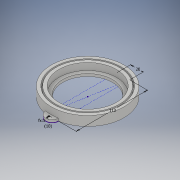
# Autodesk Inventor part: Cap
Saved by Autodesk Inventor 2018 (Build 220112000, 112)
## iProperties
Created: 2017-06-25
Part Number: Cap
Material: Generic
Document SubType Name: Modeling
Designer: Soichi
Density: 1 g/cm^3
Appearance: Default
Author: Soichi
Autodesk Inventor part; units mm, degrees
ref_plane "YZ Plane" through (0, 0, 0) normal (1, 0, 0) x (0, 1, 0)
ref_plane "XZ Plane" through (0, 0, 0) normal (0, 1, 0) x (-1, 0, 0)
ref_plane "XY Plane" through (0, 0, 0) normal (0, 0, 1) x (1, 0, 0)
sketch "Sketch1" plane through (0, 0, 0) normal (0, 0, 1) x (1, 0, 0)
  circle A0 centre (0, 0) radius 57.5
  dimension "d0" = 115
  constraints: 1 centre point, 1 coincident
  measures "d0" diameter of A0
sketch "Sketch2" plane through (0, 0, 0) normal (1, 0, 0) x (0, 1, 0)
  line L0 (57.5, 0) -> (-57.5, 0) construction
  line L1 (-57.5, 0) -> (-57.5, 15)
  line L2 (-57.5, 15) -> (-39.5, 15)
  line L3 (-39.5, 15) -> (-39.5, 11)
  line L4 (-57.5, 0) -> (-52.5, 0)
  line L5 (-52.5, 0) -> (-52.5, 8)
  line L6 (-52.5, 8) -> (-50.42, 8)
  line L7 (-50.42, 8) -> (-50.42, 0)
  line L8 (-50.42, 0) -> (-45.42, 0)
  line L9 (-50.42, 0) -> (-45.42, 0) construction
  line L10 (-45.42, 0) -> (-45.42, 11)
  line L11 (-45.42, 11) -> (-39.5, 11)
  point P0 (0, 0)
  dimension "d1" = 15
  dimension "d3" = 4
  dimension "d4" = 90
  dimension "d5" = 5
  dimension "d6" = 8
  dimension "d7" = 2.08
  dimension "d8" = 5
  dimension "d9" = 0
  dimension "d10" = 90
  dimension "d15" = 13
  constraints: 22 end point, 4 perpendicular, 3 horizontal, 2 point on line, 1 collinear, 1 parallel, 1 vertical
  measures "d1" distance of L0.end L1.end
  measures "d3" distance of L2.end L3.end
  measures "d4" angle of L2 L3
  measures "d5" distance of L0.end L4.end
  measures "d6" distance of L4.end L5.end
  measures "d7" distance of L5.end L6.end
  measures "d8" distance of L7.end L8.end
  measures "d9" distance between parallel lines of L8 L9
  measures "d10" angle of L10 L8
  measures "d15" distance between parallel lines of L3 L5
sweep "Sweep1" add profiles "Sketch2" path "Sketch1"
sketch "Sketch3" plane through (0, 0, 15) normal (0, 0, 1) x (1, 0, 0)
  line L0 (56.5, 10) -> (-56.5, 10) construction
  line L1 (-56.5, 10) -> (-56.5, -10)
  line L2 (-56.5, -10) -> (56.5, -10) construction
  line L3 (56.5, -10) -> (56.5, 10)
  line L4 (56.5, 10) -> (-56.5, -10) construction
  arc A0 (-56.5, 10) -> (-56.5, -10) centre (-56.5, 0) ccw
  arc A1 (56.5, -10) -> (56.5, 10) centre (56.5, 0) ccw
  point P0 (0, 0)
  point P1 (0, 0)
  point P2 (-61.5, 0)
  dimension "d16" = 113
  dimension "d17" = 20
  dimension "d18" = 5
  dimension "d19" = 10
  constraints: 10 end point, 4 point on circle, 3 midpoint, 2 centre point, 2 parallel, 1 coincident, 1 horizontal, 1 perpendicular
  measures "d16" distance of L0.start L0.end
  measures "d17" distance of L2.end L0.start
  measures "d18" distance of A0.centre point (-61.5, 0)
  measures "d19" radius of A0
extrude "Extrusion1" add sketch "Sketch3" against normal blind 4
hole "Hole1" at (-61.5, 0, 15) direction (0, 0, -1) diameter 3 end through all
equation "\"d18\" = 0.5 * d19"
body "Solid1"
